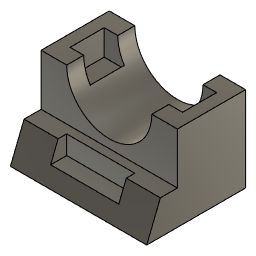
Sketch9_Final v1 (Autodesk Fusion 360 design; units mm, degrees)
Autodesk Fusion 360 part; units mm, degrees
sketch "Sketch1" plane through (0, 0, 0) normal (0, 1, 0) x (1, 0, 0)
  line L0 (0, 0) -> (40, 0)
  line L1 (40, 0) -> (40, -50)
  line L2 (40, -50) -> (25, -50)
  line L3 (0, 0) -> (-40, 0)
  line L4 (-40, 0) -> (-40, -50)
  line L5 (-40, -50) -> (-25, -50)
  arc A0 (25, -50) -> (-25, -50) centre (0, -50) ccw
  dimension "d1" = 40
  dimension "d3" = 40
  dimension "d4" = 50
  dimension "d5" = 50
  constraint horizontal L0
  constraint vertical L1
  constraint horizontal L2
  constraint coincident L0.start L3.start
  constraint horizontal L3
  constraint vertical L4
  constraint horizontal L5
  measures "d1" distance of L0.start L0.end
  measures "d3" distance of L0.start L3.end
  measures "d4" distance of L0.start A0.centre
  measures "d5" diameter of A0
extrude "Extrude1" add sketch "Sketch1" along normal blind 40
sketch "Sketch2" plane through (0, 0, 0) normal (0, 0, 1) x (1, 0, 0)
  line L0 (25, 10) -> (33, 10)
  line L1 (33, 10) -> (33, 30)
  line L2 (33, 30) -> (25, 30)
  line L3 (-33, 10) -> (-33, 30)
  line L4 (-25, 10) -> (-33, 10)
  line L5 (-33, 30) -> (-25, 30)
  line L6 (25, 10) -> (21, 10)
  line L7 (21, 10) -> (21, 30)
  line L8 (21, 30) -> (25, 30)
  line L9 (-25, 10) -> (-21.1862, 10)
  line L10 (-21.1862, 10) -> (-21.1862, 30)
  line L11 (-21.1862, 30) -> (-25, 30)
  dimension "d9" = 8
  dimension "d10" = 20
  constraint horizontal L0
  constraint vertical L1
  constraint horizontal L2
  constraint horizontal L6
  constraint vertical L7
  constraint horizontal L8
  constraint horizontal L9
  constraint vertical L10
  constraint horizontal L11
  measures "d9" distance of L0.start L0.end
  measures "d10" distance of L0.start L2.end
extrude "Extrude2" cut sketch "Sketch2" along normal blind 20 from surface at 35
sketch "Sketch4" plane through (0, 0, 0) normal (0, 1, 0) x (1, 0, 0)
  line L0 (-40, 0) -> (40, 0)
  line L1 (40, 0) -> (40, -20)
  line L2 (40, -20) -> (-40, -20)
  line L3 (-40, -20) -> (-40, 0)
  dimension "d14" = 80
  dimension "d15" = 20
  constraint horizontal L0
  constraint vertical L1
  constraint horizontal L2
  constraint vertical L3
  measures "d14" distance of L0.start L0.end
  measures "d15" distance of L0.start L2.end
extrude "Extrude3" add sketch "Sketch4" against normal blind 18
sketch "Sketch5" plane through (0, 0, 0) normal (1, 0, 0) x (0, 1, 0)
  line L0 (-18, 0) -> (-10, 20)
  line L1 (-18, 20) -> (-18, 0)
  line L2 (-18, 20) -> (-10, 20)
  constraint perpendicular L1 L2
extrude "Extrude4" cut sketch "Sketch5" along normal mid plane 122
sketch "Sketch6" plane through (0, 0, 0) normal (0, 0, 1) x (1, 0, 0)
  line L0 (20, -5) -> (-20, -5)
  line L1 (20, -5) -> (-20, 5) construction
  line L2 (-20, -5) -> (20, 5) construction
  line L3 (20, -5) -> (20, -17)
  line L4 (20, -17) -> (-20, -17)
  line L5 (-20, -17) -> (-20, -5)
  dimension "d21" = 40
  dimension "d22" = 10
  constraint horizontal L0
  constraint coincident L1 origin
  constraint coincident L2 origin
  constraint vertical L3
  constraint horizontal L4
  constraint vertical L5
  measures "d21" distance of L1.end L2.end
  measures "d22" distance of L0.end L1.end
extrude "Extrude5" cut sketch "Sketch6" along normal blind 11 from surface at 9
